Autodesk Fusion 360 part; units mm, degrees
(part 5 of 7)
  spline S32 degree 5 poles (18.221, -3.6679) (18.2206, -3.6713) (18.2199, -3.6782) (18.2192, -3.6885) (18.2187, -3.7024) (18.219, -3.7197) (18.2198, -3.7371) (18.2209, -3.7545) (18.2223, -3.7719) (18.2238, -3.7893) (18.2254, -3.8068) (18.2271, -3.8243) (18.2291, -3.8417) (18.2314, -3.8592) (18.234, -3.8768) (18.2368, -3.8943) (18.2398, -3.9118) (18.243, -3.9293) (18.2464, -3.9469) (18.2499, -3.9644) (18.2535, -3.982) (18.2574, -3.9995) (18.2614, -4.0171) (18.2655, -4.0347) (18.2699, -4.0522) (18.2744, -4.0698) (18.279, -4.0874) (18.2839, -4.1049) (18.2888, -4.1225) (18.2939, -4.1401) (18.2992, -4.1576) (18.3045, -4.1752) (18.3101, -4.1928) (18.3157, -4.2103) (18.3215, -4.2279) (18.3275, -4.2454) (18.3336, -4.2629) (18.3398, -4.2805) (18.3461, -4.298) (18.3526, -4.3155) (18.3592, -4.3331) (18.3659, -4.3506) (18.3728, -4.3681) (18.3798, -4.3856) (18.3869, -4.403) (18.3941, -4.4205) (18.4015, -4.438) (18.409, -4.4554) (18.4166, -4.4729) (18.4243, -4.4903) (18.4321, -4.5077) (18.4401, -4.5252) (18.4481, -4.5426) (18.4563, -4.5599) (18.4646, -4.5773) (18.4731, -4.5947) (18.4816, -4.612) (18.4903, -4.6293) (18.499, -4.6467) (18.5079, -4.664) (18.5169, -4.6813) (18.526, -4.6985) (18.5352, -4.7158) (18.5445, -4.733) (18.554, -4.7502) (18.5635, -4.7674) (18.5732, -4.7846) (18.5829, -4.8018) (18.5928, -4.8189) (18.6028, -4.8361) (18.6129, -4.8532) (18.621, -4.8668) (18.6272, -4.8771) (18.6313, -4.8839) (18.6334, -4.8873) knots 0 0 0 0 0 0 0.01428571 0.02857143 0.04285714 0.05714286 0.07142857 0.08571429 0.1 0.11428571 0.12857143 0.14285714 0.15714286 0.17142857 0.18571429 0.2 0.21428571 0.22857143 0.24285714 0.25714286 0.27142857 0.28571429 0.3 0.31428571 0.32857143 0.34285714 0.35714286 0.37142857 0.38571429 0.4 0.41428571 0.42857143 0.44285714 0.45714286 0.47142857 0.48571429 0.5 0.51428571 0.52857143 0.54285714 0.55714286 0.57142857 0.58571429 0.6 0.61428571 0.62857143 0.64285714 0.65714286 0.67142857 0.68571429 0.7 0.71428571 0.72857143 0.74285714 0.75714286 0.77142857 0.78571429 0.8 0.81428571 0.82857143 0.84285714 0.85714286 0.87142857 0.88571429 0.9 0.91428571 0.92857143 0.94285714 0.95714286 0.97142857 0.98571429 1 1 1 1 1 1
  arc A50 (18.6334, -4.8873) -> (19.1658, -4.8873) centre (18.8996, 2.3078) ccw
  spline S33 degree 5 poles (19.1658, -4.8873) (19.1679, -4.8839) (19.172, -4.8771) (19.1782, -4.8668) (19.1863, -4.8532) (19.1964, -4.8361) (19.2064, -4.8189) (19.2162, -4.8018) (19.226, -4.7846) (19.2356, -4.7674) (19.2452, -4.7502) (19.2546, -4.733) (19.2639, -4.7158) (19.2732, -4.6985) (19.2823, -4.6813) (19.2913, -4.664) (19.3001, -4.6467) (19.3089, -4.6293) (19.3176, -4.612) (19.3261, -4.5947) (19.3345, -4.5773) (19.3428, -4.5599) (19.351, -4.5426) (19.3591, -4.5252) (19.367, -4.5077) (19.3749, -4.4903) (19.3826, -4.4729) (19.3902, -4.4554) (19.3977, -4.438) (19.405, -4.4205) (19.4123, -4.403) (19.4194, -4.3856) (19.4264, -4.3681) (19.4332, -4.3506) (19.44, -4.3331) (19.4466, -4.3155) (19.453, -4.298) (19.4594, -4.2805) (19.4656, -4.2629) (19.4717, -4.2454) (19.4776, -4.2279) (19.4834, -4.2103) (19.4891, -4.1928) (19.4946, -4.1752) (19.5, -4.1576) (19.5052, -4.1401) (19.5103, -4.1225) (19.5153, -4.1049) (19.5201, -4.0874) (19.5248, -4.0698) (19.5293, -4.0522) (19.5336, -4.0347) (19.5378, -4.0171) (19.5418, -3.9995) (19.5456, -3.982) (19.5493, -3.9644) (19.5528, -3.9469) (19.5562, -3.9293) (19.5594, -3.9118) (19.5624, -3.8943) (19.5652, -3.8768) (19.5677, -3.8592) (19.57, -3.8417) (19.572, -3.8243) (19.5738, -3.8068) (19.5754, -3.7893) (19.5769, -3.7719) (19.5782, -3.7545) (19.5794, -3.7371) (19.5802, -3.7197) (19.5804, -3.7024) (19.58, -3.6885) (19.5793, -3.6782) (19.5786, -3.6713) (19.5782, -3.6679) knots -1 -1 -1 -1 -1 -1 -0.98571429 -0.97142857 -0.95714286 -0.94285714 -0.92857143 -0.91428571 -0.9 -0.88571429 -0.87142857 -0.85714286 -0.84285714 -0.82857143 -0.81428571 -0.8 -0.78571429 -0.77142857 -0.75714286 -0.74285714 -0.72857143 -0.71428571 -0.7 -0.68571429 -0.67142857 -0.65714286 -0.64285714 -0.62857143 -0.61428571 -0.6 -0.58571429 -0.57142857 -0.55714286 -0.54285714 -0.52857143 -0.51428571 -0.5 -0.48571429 -0.47142857 -0.45714286 -0.44285714 -0.42857143 -0.41428571 -0.4 -0.38571429 -0.37142857 -0.35714286 -0.34285714 -0.32857143 -0.31428571 -0.3 -0.28571429 -0.27142857 -0.25714286 -0.24285714 -0.22857143 -0.21428571 -0.2 -0.18571429 -0.17142857 -0.15714286 -0.14285714 -0.12857143 -0.11428571 -0.1 -0.08571429 -0.07142857 -0.05714286 -0.04285714 -0.02857143 -0.01428571 0 0 0 0 0 0
  line L50 (19.5782, -3.6679) -> (19.5395, -3.3269)
  arc A51 (19.7086, -3.1065) -> (19.5395, -3.3269) centre (19.7382, -3.3043) ccw
  line L51 (19.7086, -3.1065) -> (19.7086, -1.3065)
  line L52 (19.7086, -1.3065) -> (-29.6351, -1.3065)
  line L53 (-24.6351, -26.3065) -> (-24.6351, -3.1065)
  line L54 (-29.6351, -26.3065) -> (-24.6351, -26.3065)
  line L55 (-29.6351, -1.3065) -> (-29.6351, -26.3065)
  arc A52 (-24.466, -3.3269) -> (-24.6351, -3.1065) centre (-24.6647, -3.3043) ccw
  line L56 (-24.466, -3.3269) -> (-24.5047, -3.6679)
  spline S34 degree 5 poles (-24.5047, -3.6679) (-24.5051, -3.6713) (-24.5058, -3.6782) (-24.5065, -3.6885) (-24.5069, -3.7024) (-24.5067, -3.7197) (-24.5059, -3.7371) (-24.5047, -3.7545) (-24.5034, -3.7719) (-24.5019, -3.7893) (-24.5003, -3.8068) (-24.4985, -3.8243) (-24.4965, -3.8417) (-24.4942, -3.8592) (-24.4917, -3.8768) (-24.4889, -3.8943) (-24.4859, -3.9118) (-24.4827, -3.9293) (-24.4793, -3.9469) (-24.4758, -3.9644) (-24.4721, -3.982) (-24.4683, -3.9995) (-24.4643, -4.0171) (-24.4601, -4.0347) (-24.4558, -4.0522) (-24.4513, -4.0698) (-24.4466, -4.0874) (-24.4418, -4.1049) (-24.4368, -4.1225) (-24.4317, -4.1401) (-24.4265, -4.1576) (-24.4211, -4.1752) (-24.4156, -4.1928) (-24.4099, -4.2103) (-24.4041, -4.2279) (-24.3982, -4.2454) (-24.3921, -4.2629) (-24.3859, -4.2805) (-24.3795, -4.298) (-24.3731, -4.3155) (-24.3665, -4.3331) (-24.3597, -4.3506) (-24.3529, -4.3681) (-24.3459, -4.3856) (-24.3388, -4.403) (-24.3315, -4.4205) (-24.3242, -4.438) (-24.3167, -4.4554) (-24.3091, -4.4729) (-24.3014, -4.4903) (-24.2935, -4.5077) (-24.2856, -4.5252) (-24.2775, -4.5426) (-24.2693, -4.5599) (-24.261, -4.5773) (-24.2526, -4.5947) (-24.2441, -4.612) (-24.2354, -4.6293) (-24.2266, -4.6467) (-24.2178, -4.664) (-24.2088, -4.6813) (-24.1997, -4.6985) (-24.1904, -4.7158) (-24.1811, -4.733) (-24.1717, -4.7502) (-24.1621, -4.7674) (-24.1525, -4.7846) (-24.1427, -4.8018) (-24.1329, -4.8189) (-24.1229, -4.8361) (-24.1128, -4.8532) (-24.1047, -4.8668) (-24.0985, -4.8771) (-24.0944, -4.8839) (-24.0923, -4.8873) knots 0 0 0 0 0 0 0.01428571 0.02857143 0.04285714 0.05714286 0.07142857 0.08571429 0.1 0.11428571 0.12857143 0.14285714 0.15714286 0.17142857 0.18571429 0.2 0.21428571 0.22857143 0.24285714 0.25714286 0.27142857 0.28571429 0.3 0.31428571 0.32857143 0.34285714 0.35714286 0.37142857 0.38571429 0.4 0.41428571 0.42857143 0.44285714 0.45714286 0.47142857 0.48571429 0.5 0.51428571 0.52857143 0.54285714 0.55714286 0.57142857 0.58571429 0.6 0.61428571 0.62857143 0.64285714 0.65714286 0.67142857 0.68571429 0.7 0.71428571 0.72857143 0.74285714 0.75714286 0.77142857 0.78571429 0.8 0.81428571 0.82857143 0.84285714 0.85714286 0.87142857 0.88571429 0.9 0.91428571 0.92857143 0.94285714 0.95714286 0.97142857 0.98571429 1 1 1 1 1 1
  arc A53 (-24.0923, -4.8873) -> (-23.5599, -4.8873) centre (-23.8261, 2.3078) ccw
  spline S35 degree 5 poles (-23.5599, -4.8873) (-23.5578, -4.8839) (-23.5537, -4.8771) (-23.5475, -4.8668) (-23.5394, -4.8532) (-23.5293, -4.8361) (-23.5193, -4.8189) (-23.5094, -4.8018) (-23.4997, -4.7846) (-23.49, -4.7674) (-23.4805, -4.7502) (-23.471, -4.733) (-23.4617, -4.7158) (-23.4525, -4.6985) (-23.4434, -4.6813) (-23.4344, -4.664) (-23.4255, -4.6467) (-23.4168, -4.6293) (-23.4081, -4.612) (-23.3996, -4.5947) (-23.3911, -4.5773) (-23.3828, -4.5599) (-23.3746, -4.5426) (-23.3666, -4.5252) (-23.3586, -4.5077) (-23.3508, -4.4903) (-23.3431, -4.4729) (-23.3355, -4.4554) (-23.328, -4.438) (-23.3206, -4.4205) (-23.3134, -4.403) (-23.3063, -4.3856) (-23.2993, -4.3681) (-23.2924, -4.3506) (-23.2857, -4.3331) (-23.2791, -4.3155) (-23.2726, -4.298) (-23.2663, -4.2805) (-23.2601, -4.2629) (-23.254, -4.2454) (-23.248, -4.2279) (-23.2422, -4.2103) (-23.2366, -4.1928) (-23.231, -4.1752) (-23.2257, -4.1576) (-23.2204, -4.1401) (-23.2153, -4.1225) (-23.2104, -4.1049) (-23.2055, -4.0874) (-23.2009, -4.0698) (-23.1964, -4.0522) (-23.192, -4.0347) (-23.1879, -4.0171) (-23.1839, -3.9995) (-23.18, -3.982) (-23.1764, -3.9644) (-23.1729, -3.9469) (-23.1695, -3.9293) (-23.1663, -3.9118) (-23.1633, -3.8943) (-23.1605, -3.8768) (-23.1579, -3.8592) (-23.1556, -3.8417) (-23.1536, -3.8243) (-23.1519, -3.8068) (-23.1503, -3.7893) (-23.1488, -3.7719) (-23.1474, -3.7545) (-23.1463, -3.7371) (-23.1455, -3.7197) (-23.1452, -3.7024) (-23.1457, -3.6885) (-23.1464, -3.6782) (-23.1471, -3.6713) (-23.1475, -3.6679) knots -1 -1 -1 -1 -1 -1 -0.98571429 -0.97142857 -0.95714286 -0.94285714 -0.92857143 -0.91428571 -0.9 -0.88571429 -0.87142857 -0.85714286 -0.84285714 -0.82857143 -0.81428571 -0.8 -0.78571429 -0.77142857 -0.75714286 -0.74285714 -0.72857143 -0.71428571 -0.7 -0.68571429 -0.67142857 -0.65714286 -0.64285714 -0.62857143 -0.61428571 -0.6 -0.58571429 -0.57142857 -0.55714286 -0.54285714 -0.52857143 -0.51428571 -0.5 -0.48571429 -0.47142857 -0.45714286 -0.44285714 -0.42857143 -0.41428571 -0.4 -0.38571429 -0.37142857 -0.35714286 -0.34285714 -0.32857143 -0.31428571 -0.3 -0.28571429 -0.27142857 -0.25714286 -0.24285714 -0.22857143 -0.21428571 -0.2 -0.18571429 -0.17142857 -0.15714286 -0.14285714 -0.12857143 -0.11428571 -0.1 -0.08571429 -0.07142857 -0.05714286 -0.04285714 -0.02857143 -0.01428571 0 0 0 0 0 0
  line L57 (-23.1475, -3.6679) -> (-23.1862, -3.3269)
  line L58 (-24.6351, -3.1065) -> (-29.6351, -3.1065)
  constraint coincident L53.end A52.end
  constraint coincident L55 L58.end
  constraint perpendicular L55 L58
extrude "Extrude11" cut 1 faces at (27.9685, 26.3065, 2.0595) along direction (0, -1, 0) blind 10 on bodies 20 bodies 20
extrude "Extrude12" cut 1 faces at (27.9685, 16.3065, 2.0595) along direction (0, -1, 0) blind 2 on bodies 20 bodies 20
sketch "Sketch13" plane through (0, 0, 3.3929) normal (0, 0, 1) x (-1, 0, 0)
  line L0 (-29.6351, -14.3065) -> (-24.6351, -14.3065)
  line L1 (-24.6351, -14.3065) -> (-24.6351, -3.1065)
  arc A0 (-24.466, -3.3269) -> (-24.6351, -3.1065) centre (-24.6647, -3.3043) ccw
  line L2 (-24.466, -3.3269) -> (-24.5047, -3.6679)
  spline S0 degree 5 poles (-24.5047, -3.6679) (-24.5051, -3.6713) (-24.5058, -3.6782) (-24.5065, -3.6885) (-24.5069, -3.7024) (-24.5067, -3.7197) (-24.5059, -3.7371) (-24.5047, -3.7545) (-24.5034, -3.7719) (-24.5019, -3.7893) (-24.5003, -3.8068) (-24.4985, -3.8243) (-24.4965, -3.8417) (-24.4942, -3.8592) (-24.4917, -3.8768) (-24.4889, -3.8943) (-24.4859, -3.9118) (-24.4827, -3.9293) (-24.4793, -3.9469) (-24.4758, -3.9644) (-24.4721, -3.982) (-24.4683, -3.9995) (-24.4643, -4.0171) (-24.4601, -4.0347) (-24.4558, -4.0522) (-24.4513, -4.0698) (-24.4466, -4.0874) (-24.4418, -4.1049) (-24.4368, -4.1225) (-24.4317, -4.1401) (-24.4265, -4.1576) (-24.4211, -4.1752) (-24.4156, -4.1928) (-24.4099, -4.2103) (-24.4041, -4.2279) (-24.3982, -4.2454) (-24.3921, -4.2629) (-24.3859, -4.2805) (-24.3795, -4.298) (-24.3731, -4.3155) (-24.3665, -4.3331) (-24.3597, -4.3506) (-24.3529, -4.3681) (-24.3459, -4.3856) (-24.3388, -4.403) (-24.3315, -4.4205) (-24.3242, -4.438) (-24.3167, -4.4554) (-24.3091, -4.4729) (-24.3014, -4.4903) (-24.2935, -4.5077) (-24.2856, -4.5252) (-24.2775, -4.5426) (-24.2693, -4.5599) (-24.261, -4.5773) (-24.2526, -4.5947) (-24.2441, -4.612) (-24.2354, -4.6293) (-24.2266, -4.6467) (-24.2178, -4.664) (-24.2088, -4.6813) (-24.1997, -4.6985) (-24.1904, -4.7158) (-24.1811, -4.733) (-24.1717, -4.7502) (-24.1621, -4.7674) (-24.1525, -4.7846) (-24.1427, -4.8018) (-24.1329, -4.8189) (-24.1229, -4.8361) (-24.1128, -4.8532) (-24.1047, -4.8668) (-24.0985, -4.8771) (-24.0944, -4.8839) (-24.0923, -4.8873) knots 0 0 0 0 0 0 0.01428571 0.02857143 0.04285714 0.05714286 0.07142857 0.08571429 0.1 0.11428571 0.12857143 0.14285714 0.15714286 0.17142857 0.18571429 0.2 0.21428571 0.22857143 0.24285714 0.25714286 0.27142857 0.28571429 0.3 0.31428571 0.32857143 0.34285714 0.35714286 0.37142857 0.38571429 0.4 0.41428571 0.42857143 0.44285714 0.45714286 0.47142857 0.48571429 0.5 0.51428571 0.52857143 0.54285714 0.55714286 0.57142857 0.58571429 0.6 0.61428571 0.62857143 0.64285714 0.65714286 0.67142857 0.68571429 0.7 0.71428571 0.72857143 0.74285714 0.75714286 0.77142857 0.78571429 0.8 0.81428571 0.82857143 0.84285714 0.85714286 0.87142857 0.88571429 0.9 0.91428571 0.92857143 0.94285714 0.95714286 0.97142857 0.98571429 1 1 1 1 1 1
  arc A1 (-24.0923, -4.8873) -> (-23.5599, -4.8873) centre (-23.8261, 2.3078) ccw
  spline S1 degree 5 poles (-23.5599, -4.8873) (-23.5578, -4.8839) (-23.5537, -4.8771) (-23.5475, -4.8668) (-23.5394, -4.8532) (-23.5293, -4.8361) (-23.5193, -4.8189) (-23.5094, -4.8018) (-23.4997, -4.7846) (-23.49, -4.7674) (-23.4805, -4.7502) (-23.471, -4.733) (-23.4617, -4.7158) (-23.4525, -4.6985) (-23.4434, -4.6813) (-23.4344, -4.664) (-23.4255, -4.6467) (-23.4168, -4.6293) (-23.4081, -4.612) (-23.3996, -4.5947) (-23.3911, -4.5773) (-23.3828, -4.5599) (-23.3746, -4.5426) (-23.3666, -4.5252) (-23.3586, -4.5077) (-23.3508, -4.4903) (-23.3431, -4.4729) (-23.3355, -4.4554) (-23.328, -4.438) (-23.3206, -4.4205) (-23.3134, -4.403) (-23.3063, -4.3856) (-23.2993, -4.3681) (-23.2924, -4.3506) (-23.2857, -4.3331) (-23.2791, -4.3155) (-23.2726, -4.298) (-23.2663, -4.2805) (-23.2601, -4.2629) (-23.254, -4.2454) (-23.248, -4.2279) (-23.2422, -4.2103) (-23.2366, -4.1928) (-23.231, -4.1752) (-23.2257, -4.1576) (-23.2204, -4.1401) (-23.2153, -4.1225) (-23.2104, -4.1049) (-23.2055, -4.0874) (-23.2009, -4.0698) (-23.1964, -4.0522) (-23.192, -4.0347) (-23.1879, -4.0171) (-23.1839, -3.9995) (-23.18, -3.982) (-23.1764, -3.9644) (-23.1729, -3.9469) (-23.1695, -3.9293) (-23.1663, -3.9118) (-23.1633, -3.8943) (-23.1605, -3.8768) (-23.1579, -3.8592) (-23.1556, -3.8417) (-23.1536, -3.8243) (-23.1519, -3.8068) (-23.1503, -3.7893) (-23.1488, -3.7719) (-23.1474, -3.7545) (-23.1463, -3.7371) (-23.1455, -3.7197) (-23.1452, -3.7024) (-23.1457, -3.6885) (-23.1464, -3.6782) (-23.1471, -3.6713) (-23.1475, -3.6679) knots -1 -1 -1 -1 -1 -1 -0.98571429 -0.97142857 -0.95714286 -0.94285714 -0.92857143 -0.91428571 -0.9 -0.88571429 -0.87142857 -0.85714286 -0.84285714 -0.82857143 -0.81428571 -0.8 -0.78571429 -0.77142857 -0.75714286 -0.74285714 -0.72857143 -0.71428571 -0.7 -0.68571429 -0.67142857 -0.65714286 -0.64285714 -0.62857143 -0.61428571 -0.6 -0.58571429 -0.57142857 -0.55714286 -0.54285714 -0.52857143 -0.51428571 -0.5 -0.48571429 -0.47142857 -0.45714286 -0.44285714 -0.42857143 -0.41428571 -0.4 -0.38571429 -0.37142857 -0.35714286 -0.34285714 -0.32857143 -0.31428571 -0.3 -0.28571429 -0.27142857 -0.25714286 -0.24285714 -0.22857143 -0.21428571 -0.2 -0.18571429 -0.17142857 -0.15714286 -0.14285714 -0.12857143 -0.11428571 -0.1 -0.08571429 -0.07142857 -0.05714286 -0.04285714 -0.02857143 -0.01428571 0 0 0 0 0 0
  line L3 (-23.1475, -3.6679) -> (-23.1862, -3.3269)
  arc A2 (-23.017, -3.1065) -> (-23.1862, -3.3269) centre (-22.9875, -3.3043) ccw
  line L4 (-23.017, -3.1065) -> (-22.1219, -3.1065)
  arc A3 (-21.9527, -3.3269) -> (-22.1219, -3.1065) centre (-22.1514, -3.3043) ccw
  line L5 (-21.9527, -3.3269) -> (-21.9914, -3.6679)
  spline S2 degree 5 poles (-21.9914, -3.6679) (-21.9918, -3.6713) (-21.9925, -3.6782) (-21.9932, -3.6885) (-21.9936, -3.7024) (-21.9934, -3.7197) (-21.9926, -3.7371) (-21.9914, -3.7545) (-21.9901, -3.7719) (-21.9886, -3.7893) (-21.987, -3.8068) (-21.9852, -3.8243) (-21.9832, -3.8417) (-21.981, -3.8592) (-21.9784, -3.8768) (-21.9756, -3.8943) (-21.9726, -3.9118) (-21.9694, -3.9293) (-21.966, -3.9469) (-21.9625, -3.9644) (-21.9588, -3.982) (-21.955, -3.9995) (-21.951, -4.0171) (-21.9469, -4.0347) (-21.9425, -4.0522) (-21.938, -4.0698) (-21.9333, -4.0874) (-21.9285, -4.1049) (-21.9236, -4.1225) (-21.9185, -4.1401) (-21.9132, -4.1576) (-21.9078, -4.1752) (-21.9023, -4.1928) (-21.8966, -4.2103) (-21.8908, -4.2279) (-21.8849, -4.2454) (-21.8788, -4.2629) (-21.8726, -4.2805) (-21.8663, -4.298) (-21.8598, -4.3155) (-21.8532, -4.3331) (-21.8465, -4.3506) (-21.8396, -4.3681) (-21.8326, -4.3856) (-21.8255, -4.403) (-21.8183, -4.4205) (-21.8109, -4.438) (-21.8034, -4.4554) (-21.7958, -4.4729) (-21.7881, -4.4903) (-21.7803, -4.5077) (-21.7723, -4.5252) (-21.7642, -4.5426) (-21.7561, -4.5599) (-21.7477, -4.5773) (-21.7393, -4.5947) (-21.7308, -4.612) (-21.7221, -4.6293) (-21.7134, -4.6467) (-21.7045, -4.664) (-21.6955, -4.6813) (-21.6864, -4.6985) (-21.6772, -4.7158) (-21.6678, -4.733) (-21.6584, -4.7502) (-21.6489, -4.7674) (-21.6392, -4.7846) (-21.6295, -4.8018) (-21.6196, -4.8189) (-21.6096, -4.8361) (-21.5995, -4.8532) (-21.5914, -4.8668) (-21.5852, -4.8771) (-21.5811, -4.8839) (-21.579, -4.8873) knots 0 0 0 0 0 0 0.01428571 0.02857143 0.04285714 0.05714286 0.07142857 0.08571429 0.1 0.11428571 0.12857143 0.14285714 0.15714286 0.17142857 0.18571429 0.2 0.21428571 0.22857143 0.24285714 0.25714286 0.27142857 0.28571429 0.3 0.31428571 0.32857143 0.34285714 0.35714286 0.37142857 0.38571429 0.4 0.41428571 0.42857143 0.44285714 0.45714286 0.47142857 0.48571429 0.5 0.51428571 0.52857143 0.54285714 0.55714286 0.57142857 0.58571429 0.6 0.61428571 0.62857143 0.64285714 0.65714286 0.67142857 0.68571429 0.7 0.71428571 0.72857143 0.74285714 0.75714286 0.77142857 0.78571429 0.8 0.81428571 0.82857143 0.84285714 0.85714286 0.87142857 0.88571429 0.9 0.91428571 0.92857143 0.94285714 0.95714286 0.97142857 0.98571429 1 1 1 1 1 1
  arc A4 (-21.579, -4.8873) -> (-21.0466, -4.8873) centre (-21.3128, 2.3078) ccw
  spline S3 degree 5 poles (-21.0466, -4.8873) (-21.0445, -4.8839) (-21.0404, -4.8771) (-21.0342, -4.8668) (-21.0261, -4.8532) (-21.016, -4.8361) (-21.006, -4.8189) (-20.9962, -4.8018) (-20.9864, -4.7846) (-20.9767, -4.7674) (-20.9672, -4.7502) (-20.9578, -4.733) (-20.9484, -4.7158) (-20.9392, -4.6985) (-20.9301, -4.6813) (-20.9211, -4.664) (-20.9123, -4.6467) (-20.9035, -4.6293) (-20.8948, -4.612) (-20.8863, -4.5947) (-20.8779, -4.5773) (-20.8696, -4.5599) (-20.8614, -4.5426) (-20.8533, -4.5252) (-20.8453, -4.5077) (-20.8375, -4.4903) (-20.8298, -4.4729) (-20.8222, -4.4554) (-20.8147, -4.438) (-20.8073, -4.4205) (-20.8001, -4.403) (-20.793, -4.3856) (-20.786, -4.3681) (-20.7792, -4.3506) (-20.7724, -4.3331) (-20.7658, -4.3155) (-20.7594, -4.298) (-20.753, -4.2805) (-20.7468, -4.2629) (-20.7407, -4.2454) (-20.7348, -4.2279) (-20.729, -4.2103) (-20.7233, -4.1928) (-20.7178, -4.1752) (-20.7124, -4.1576) (-20.7071, -4.1401) (-20.702, -4.1225) (-20.6971, -4.1049) (-20.6923, -4.0874) (-20.6876, -4.0698) (-20.6831, -4.0522) (-20.6788, -4.0347) (-20.6746, -4.0171) (-20.6706, -3.9995) (-20.6668, -3.982) (-20.6631, -3.9644) (-20.6596, -3.9469) (-20.6562, -3.9293) (-20.653, -3.9118) (-20.65, -3.8943) (-20.6472, -3.8768) (-20.6446, -3.8592) (-20.6424, -3.8417) (-20.6404, -3.8243) (-20.6386, -3.8068) (-20.637, -3.7893) (-20.6355, -3.7719) (-20.6342, -3.7545) (-20.633, -3.7371) (-20.6322, -3.7197) (-20.632, -3.7024) (-20.6324, -3.6885) (-20.6331, -3.6782) (-20.6338, -3.6713) (-20.6342, -3.6679) knots -1 -1 -1 -1 -1 -1 -0.98571429 -0.97142857 -0.95714286 -0.94285714 -0.92857143 -0.91428571 -0.9 -0.88571429 -0.87142857 -0.85714286 -0.84285714 -0.82857143 -0.81428571 -0.8 -0.78571429 -0.77142857 -0.75714286 -0.74285714 -0.72857143 -0.71428571 -0.7 -0.68571429 -0.67142857 -0.65714286 -0.64285714 -0.62857143 -0.61428571 -0.6 -0.58571429 -0.57142857 -0.55714286 -0.54285714 -0.52857143 -0.51428571 -0.5 -0.48571429 -0.47142857 -0.45714286 -0.44285714 -0.42857143 -0.41428571 -0.4 -0.38571429 -0.37142857 -0.35714286 -0.34285714 -0.32857143 -0.31428571 -0.3 -0.28571429 -0.27142857 -0.25714286 -0.24285714 -0.22857143 -0.21428571 -0.2 -0.18571429 -0.17142857 -0.15714286 -0.14285714 -0.12857143 -0.11428571 -0.1 -0.08571429 -0.07142857 -0.05714286 -0.04285714 -0.02857143 -0.01428571 0 0 0 0 0 0
  line L6 (-20.6342, -3.6679) -> (-20.6729, -3.3269)
  arc A5 (-20.5037, -3.1065) -> (-20.6729, -3.3269) centre (-20.4742, -3.3043) ccw
  line L7 (-20.5037, -3.1065) -> (-19.6086, -3.1065)
  arc A6 (-19.4394, -3.3269) -> (-19.6086, -3.1065) centre (-19.6381, -3.3043) ccw
  line L8 (-19.4394, -3.3269) -> (-19.4781, -3.6679)
  spline S4 degree 5 poles (-19.4781, -3.6679) (-19.4785, -3.6713) (-19.4792, -3.6782) (-19.48, -3.6885) (-19.4804, -3.7024) (-19.4801, -3.7197) (-19.4793, -3.7371) (-19.4782, -3.7545) (-19.4768, -3.7719) (-19.4753, -3.7893) (-19.4737, -3.8068) (-19.472, -3.8243) (-19.47, -3.8417) (-19.4677, -3.8592) (-19.4652, -3.8768) (-19.4624, -3.8943) (-19.4593, -3.9118) (-19.4561, -3.9293) (-19.4528, -3.9469) (-19.4492, -3.9644) (-19.4456, -3.982) (-19.4417, -3.9995) (-19.4377, -4.0171) (-19.4336, -4.0347) (-19.4292, -4.0522) (-19.4247, -4.0698) (-19.4201, -4.0874) (-19.4153, -4.1049) (-19.4103, -4.1225) (-19.4052, -4.1401) (-19.4, -4.1576) (-19.3946, -4.1752) (-19.389, -4.1928) (-19.3834, -4.2103) (-19.3776, -4.2279) (-19.3716, -4.2454) (-19.3655, -4.2629) (-19.3593, -4.2805) (-19.353, -4.298) (-19.3465, -4.3155) (-19.3399, -4.3331) (-19.3332, -4.3506) (-19.3263, -4.3681) (-19.3193, -4.3856) (-19.3122, -4.403) (-19.305, -4.4205) (-19.2976, -4.438) (-19.2902, -4.4554) (-19.2826, -4.4729) (-19.2748, -4.4903) (-19.267, -4.5077) (-19.259, -4.5252) (-19.251, -4.5426) (-19.2428, -4.5599) (-19.2345, -4.5773) (-19.226, -4.5947) (-19.2175, -4.612) (-19.2089, -4.6293) (-19.2001, -4.6467) (-19.1912, -4.664) (-19.1822, -4.6813) (-19.1731, -4.6985) (-19.1639, -4.7158) (-19.1546, -4.733) (-19.1451, -4.7502) (-19.1356, -4.7674) (-19.1259, -4.7846) (-19.1162, -4.8018) (-19.1063, -4.8189) (-19.0963, -4.8361) (-19.0863, -4.8532) (-19.0781, -4.8668) (-19.072, -4.8771) (-19.0678, -4.8839) (-19.0658, -4.8873) knots 0 0 0 0 0 0 0.01428571 0.02857143 0.04285714 0.05714286 0.07142857 0.08571429 0.1 0.11428571 0.12857143 0.14285714 0.15714286 0.17142857 0.18571429 0.2 0.21428571 0.22857143 0.24285714 0.25714286 0.27142857 0.28571429 0.3 0.31428571 0.32857143 0.34285714 0.35714286 0.37142857 0.38571429 0.4 0.41428571 0.42857143 0.44285714 0.45714286 0.47142857 0.48571429 0.5 0.51428571 0.52857143 0.54285714 0.55714286 0.57142857 0.58571429 0.6 0.61428571 0.62857143 0.64285714 0.65714286 0.67142857 0.68571429 0.7 0.71428571 0.72857143 0.74285714 0.75714286 0.77142857 0.78571429 0.8 0.81428571 0.82857143 0.84285714 0.85714286 0.87142857 0.88571429 0.9 0.91428571 0.92857143 0.94285714 0.95714286 0.97142857 0.98571429 1 1 1 1 1 1
  arc A7 (-19.0658, -4.8873) -> (-18.5333, -4.8873) centre (-18.7995, 2.3078) ccw
  spline S5 degree 5 poles (-18.5333, -4.8873) (-18.5312, -4.8839) (-18.5271, -4.8771) (-18.521, -4.8668) (-18.5128, -4.8532) (-18.5027, -4.8361) (-18.4927, -4.8189) (-18.4829, -4.8018) (-18.4731, -4.7846) (-18.4635, -4.7674) (-18.4539, -4.7502) (-18.4445, -4.733) (-18.4352, -4.7158) (-18.426, -4.6985) (-18.4168, -4.6813) (-18.4079, -4.664) (-18.399, -4.6467) (-18.3902, -4.6293) (-18.3816, -4.612) (-18.373, -4.5947) (-18.3646, -4.5773) (-18.3563, -4.5599) (-18.3481, -4.5426) (-18.34, -4.5252) (-18.3321, -4.5077) (-18.3242, -4.4903) (-18.3165, -4.4729) (-18.3089, -4.4554) (-18.3014, -4.438) (-18.2941, -4.4205) (-18.2868, -4.403) (-18.2797, -4.3856) (-18.2727, -4.3681) (-18.2659, -4.3506) (-18.2592, -4.3331) (-18.2526, -4.3155) (-18.2461, -4.298) (-18.2397, -4.2805) (-18.2335, -4.2629) (-18.2274, -4.2454) (-18.2215, -4.2279) (-18.2157, -4.2103) (-18.21, -4.1928) (-18.2045, -4.1752) (-18.1991, -4.1576) (-18.1939, -4.1401) (-18.1888, -4.1225) (-18.1838, -4.1049) (-18.179, -4.0874) (-18.1743, -4.0698) (-18.1698, -4.0522) (-18.1655, -4.0347) (-18.1613, -4.0171) (-18.1573, -3.9995) (-18.1535, -3.982) (-18.1498, -3.9644) (-18.1463, -3.9469) (-18.1429, -3.9293) (-18.1397, -3.9118) (-18.1367, -3.8943) (-18.1339, -3.8768) (-18.1314, -3.8592) (-18.1291, -3.8417) (-18.1271, -3.8243) (-18.1253, -3.8068) (-18.1237, -3.7893) (-18.1222, -3.7719) (-18.1209, -3.7545) (-18.1197, -3.7371) (-18.1189, -3.7197) (-18.1187, -3.7024) (-18.1191, -3.6885) (-18.1198, -3.6782) (-18.1205, -3.6713) (-18.1209, -3.6679) knots -1 -1 -1 -1 -1 -1 -0.98571429 -0.97142857 -0.95714286 -0.94285714 -0.92857143 -0.91428571 -0.9 -0.88571429 -0.87142857 -0.85714286 -0.84285714 -0.82857143 -0.81428571 -0.8 -0.78571429 -0.77142857 -0.75714286 -0.74285714 -0.72857143 -0.71428571 -0.7 -0.68571429 -0.67142857 -0.65714286 -0.64285714 -0.62857143 -0.61428571 -0.6 -0.58571429 -0.57142857 -0.55714286 -0.54285714 -0.52857143 -0.51428571 -0.5 -0.48571429 -0.47142857 -0.45714286 -0.44285714 -0.42857143 -0.41428571 -0.4 -0.38571429 -0.37142857 -0.35714286 -0.34285714 -0.32857143 -0.31428571 -0.3 -0.28571429 -0.27142857 -0.25714286 -0.24285714 -0.22857143 -0.21428571 -0.2 -0.18571429 -0.17142857 -0.15714286 -0.14285714 -0.12857143 -0.11428571 -0.1 -0.08571429 -0.07142857 -0.05714286 -0.04285714 -0.02857143 -0.01428571 0 0 0 0 0 0
  line L9 (-18.1209, -3.6679) -> (-18.1596, -3.3269)
  arc A8 (-17.9905, -3.1065) -> (-18.1596, -3.3269) centre (-17.9609, -3.3043) ccw
  line L10 (-17.9905, -3.1065) -> (-17.0953, -3.1065)
  arc A9 (-16.9262, -3.3269) -> (-17.0953, -3.1065) centre (-17.1249, -3.3043) ccw
  line L11 (-16.9262, -3.3269) -> (-16.9649, -3.6679)
  spline S6 degree 5 poles (-16.9649, -3.6679) (-16.9653, -3.6713) (-16.9659, -3.6782) (-16.9667, -3.6885) (-16.9671, -3.7024) (-16.9668, -3.7197) (-16.966, -3.7371) (-16.9649, -3.7545) (-16.9635, -3.7719) (-16.9621, -3.7893) (-16.9605, -3.8068) (-16.9587, -3.8243) (-16.9567, -3.8417) (-16.9544, -3.8592) (-16.9519, -3.8768) (-16.9491, -3.8943) (-16.9461, -3.9118) (-16.9429, -3.9293) (-16.9395, -3.9469) (-16.936, -3.9644) (-16.9323, -3.982) (-16.9285, -3.9995) (-16.9245, -4.0171) (-16.9203, -4.0347) (-16.916, -4.0522) (-16.9115, -4.0698) (-16.9068, -4.0874) (-16.902, -4.1049) (-16.897, -4.1225) (-16.8919, -4.1401) (-16.8867, -4.1576) (-16.8813, -4.1752) (-16.8758, -4.1928) (-16.8701, -4.2103) (-16.8643, -4.2279) (-16.8583, -4.2454) (-16.8523, -4.2629) (-16.8461, -4.2805) (-16.8397, -4.298) (-16.8332, -4.3155) (-16.8266, -4.3331) (-16.8199, -4.3506) (-16.813, -4.3681) (-16.8061, -4.3856) (-16.799, -4.403) (-16.7917, -4.4205) (-16.7844, -4.438) (-16.7769, -4.4554) (-16.7693, -4.4729) (-16.7616, -4.4903) (-16.7537, -4.5077) (-16.7458, -4.5252) (-16.7377, -4.5426) (-16.7295, -4.5599) (-16.7212, -4.5773) (-16.7128, -4.5947) (-16.7042, -4.612) (-16.6956, -4.6293) (-16.6868, -4.6467) (-16.6779, -4.664) (-16.6689, -4.6813) (-16.6598, -4.6985) (-16.6506, -4.7158) (-16.6413, -4.733) (-16.6319, -4.7502) (-16.6223, -4.7674) (-16.6127, -4.7846) (-16.6029, -4.8018) (-16.593, -4.8189) (-16.5831, -4.8361) (-16.573, -4.8532) (-16.5648, -4.8668) (-16.5587, -4.8771) (-16.5545, -4.8839) (-16.5525, -4.8873) knots 0 0 0 0 0 0 0.01428571 0.02857143 0.04285714 0.05714286 0.07142857 0.08571429 0.1 0.11428571 0.12857143 0.14285714 0.15714286 0.17142857 0.18571429 0.2 0.21428571 0.22857143 0.24285714 0.25714286 0.27142857 0.28571429 0.3 0.31428571 0.32857143 0.34285714 0.35714286 0.37142857 0.38571429 0.4 0.41428571 0.42857143 0.44285714 0.45714286 0.47142857 0.48571429 0.5 0.51428571 0.52857143 0.54285714 0.55714286 0.57142857 0.58571429 0.6 0.61428571 0.62857143 0.64285714 0.65714286 0.67142857 0.68571429 0.7 0.71428571 0.72857143 0.74285714 0.75714286 0.77142857 0.78571429 0.8 0.81428571 0.82857143 0.84285714 0.85714286 0.87142857 0.88571429 0.9 0.91428571 0.92857143 0.94285714 0.95714286 0.97142857 0.98571429 1 1 1 1 1 1
  arc A10 (-16.5525, -4.8873) -> (-16.02, -4.8873) centre (-16.2863, 2.3078) ccw
  spline S7 degree 5 poles (-16.02, -4.8873) (-16.018, -4.8839) (-16.0138, -4.8771) (-16.0077, -4.8668) (-15.9995, -4.8532) (-15.9894, -4.8361) (-15.9795, -4.8189) (-15.9696, -4.8018) (-15.9598, -4.7846) (-15.9502, -4.7674) (-15.9407, -4.7502) (-15.9312, -4.733) (-15.9219, -4.7158) (-15.9127, -4.6985) (-15.9036, -4.6813) (-15.8946, -4.664) (-15.8857, -4.6467) (-15.8769, -4.6293) (-15.8683, -4.612) (-15.8597, -4.5947) (-15.8513, -4.5773) (-15.843, -4.5599) (-15.8348, -4.5426) (-15.8267, -4.5252) (-15.8188, -4.5077) (-15.811, -4.4903) (-15.8032, -4.4729) (-15.7956, -4.4554) (-15.7882, -4.438) (-15.7808, -4.4205) (-15.7736, -4.403) (-15.7665, -4.3856) (-15.7595, -4.3681) (-15.7526, -4.3506) (-15.7459, -4.3331) (-15.7393, -4.3155) (-15.7328, -4.298) (-15.7265, -4.2805) (-15.7202, -4.2629) (-15.7142, -4.2454) (-15.7082, -4.2279) (-15.7024, -4.2103) (-15.6967, -4.1928) (-15.6912, -4.1752) (-15.6858, -4.1576) (-15.6806, -4.1401) (-15.6755, -4.1225) (-15.6705, -4.1049) (-15.6657, -4.0874) (-15.6611, -4.0698) (-15.6565, -4.0522) (-15.6522, -4.0347) (-15.648, -4.0171) (-15.644, -3.9995) (-15.6402, -3.982) (-15.6365, -3.9644) (-15.633, -3.9469) (-15.6297, -3.9293) (-15.6265, -3.9118) (-15.6234, -3.8943) (-15.6206, -3.8768) (-15.6181, -3.8592) (-15.6158, -3.8417) (-15.6138, -3.8243) (-15.612, -3.8068) (-15.6104, -3.7893) (-15.609, -3.7719) (-15.6076, -3.7545) (-15.6065, -3.7371) (-15.6057, -3.7197) (-15.6054, -3.7024) (-15.6058, -3.6885) (-15.6066, -3.6782) (-15.6073, -3.6713) (-15.6076, -3.6679) knots -1 -1 -1 -1 -1 -1 -0.98571429 -0.97142857 -0.95714286 -0.94285714 -0.92857143 -0.91428571 -0.9 -0.88571429 -0.87142857 -0.85714286 -0.84285714 -0.82857143 -0.81428571 -0.8 -0.78571429 -0.77142857 -0.75714286 -0.74285714 -0.72857143 -0.71428571 -0.7 -0.68571429 -0.67142857 -0.65714286 -0.64285714 -0.62857143 -0.61428571 -0.6 -0.58571429 -0.57142857 -0.55714286 -0.54285714 -0.52857143 -0.51428571 -0.5 -0.48571429 -0.47142857 -0.45714286 -0.44285714 -0.42857143 -0.41428571 -0.4 -0.38571429 -0.37142857 -0.35714286 -0.34285714 -0.32857143 -0.31428571 -0.3 -0.28571429 -0.27142857 -0.25714286 -0.24285714 -0.22857143 -0.21428571 -0.2 -0.18571429 -0.17142857 -0.15714286 -0.14285714 -0.12857143 -0.11428571 -0.1 -0.08571429 -0.07142857 -0.05714286 -0.04285714 -0.02857143 -0.01428571 0 0 0 0 0 0
  line L12 (-15.6076, -3.6679) -> (-15.6464, -3.3269)
  arc A11 (-15.4772, -3.1065) -> (-15.6464, -3.3269) centre (-15.4476, -3.3043) ccw
  line L13 (-15.4772, -3.1065) -> (-14.582, -3.1065)
  arc A12 (-14.4129, -3.3269) -> (-14.582, -3.1065) centre (-14.6116, -3.3043) ccw
  line L14 (-14.4129, -3.3269) -> (-14.4516, -3.6679)
  spline S8 degree 5 poles (-14.4516, -3.6679) (-14.452, -3.6713) (-14.4527, -3.6782) (-14.4534, -3.6885) (-14.4538, -3.7024) (-14.4536, -3.7197) (-14.4528, -3.7371) (-14.4516, -3.7545) (-14.4503, -3.7719) (-14.4488, -3.7893) (-14.4472, -3.8068) (-14.4454, -3.8243) (-14.4434, -3.8417) (-14.4411, -3.8592) (-14.4386, -3.8768) (-14.4358, -3.8943) (-14.4328, -3.9118) (-14.4296, -3.9293) (-14.4262, -3.9469) (-14.4227, -3.9644) (-14.419, -3.982) (-14.4152, -3.9995) (-14.4112, -4.0171) (-14.407, -4.0347) (-14.4027, -4.0522) (-14.3982, -4.0698) (-14.3935, -4.0874) (-14.3887, -4.1049) (-14.3837, -4.1225) (-14.3786, -4.1401) (-14.3734, -4.1576) (-14.368, -4.1752) (-14.3625, -4.1928) (-14.3568, -4.2103) (-14.351, -4.2279) (-14.3451, -4.2454) (-14.339, -4.2629) (-14.3328, -4.2805) (-14.3264, -4.298) (-14.32, -4.3155) (-14.3134, -4.3331) (-14.3066, -4.3506) (-14.2998, -4.3681) (-14.2928, -4.3856) (-14.2857, -4.403) (-14.2784, -4.4205) (-14.2711, -4.438) (-14.2636, -4.4554) (-14.256, -4.4729) (-14.2483, -4.4903) (-14.2405, -4.5077) (-14.2325, -4.5252) (-14.2244, -4.5426) (-14.2162, -4.5599) (-14.2079, -4.5773) (-14.1995, -4.5947) (-14.191, -4.612) (-14.1823, -4.6293) (-14.1735, -4.6467) (-14.1647, -4.664) (-14.1557, -4.6813) (-14.1466, -4.6985) (-14.1374, -4.7158) (-14.128, -4.733) (-14.1186, -4.7502) (-14.109, -4.7674) (-14.0994, -4.7846) (-14.0896, -4.8018) (-14.0798, -4.8189) (-14.0698, -4.8361) (-14.0597, -4.8532) (-14.0516, -4.8668) (-14.0454, -4.8771) (-14.0413, -4.8839) (-14.0392, -4.8873) knots 0 0 0 0 0 0 0.01428571 0.02857143 0.04285714 0.05714286 0.07142857 0.08571429 0.1 0.11428571 0.12857143 0.14285714 0.15714286 0.17142857 0.18571429 0.2 0.21428571 0.22857143 0.24285714 0.25714286 0.27142857 0.28571429 0.3 0.31428571 0.32857143 0.34285714 0.35714286 0.37142857 0.38571429 0.4 0.41428571 0.42857143 0.44285714 0.45714286 0.47142857 0.48571429 0.5 0.51428571 0.52857143 0.54285714 0.55714286 0.57142857 0.58571429 0.6 0.61428571 0.62857143 0.64285714 0.65714286 0.67142857 0.68571429 0.7 0.71428571 0.72857143 0.74285714 0.75714286 0.77142857 0.78571429 0.8 0.81428571 0.82857143 0.84285714 0.85714286 0.87142857 0.88571429 0.9 0.91428571 0.92857143 0.94285714 0.95714286 0.97142857 0.98571429 1 1 1 1 1 1
  arc A13 (-14.0392, -4.8873) -> (-13.5068, -4.8873) centre (-13.773, 2.3078) ccw
  spline S9 degree 5 poles (-13.5068, -4.8873) (-13.5047, -4.8839) (-13.5006, -4.8771) (-13.4944, -4.8668) (-13.4863, -4.8532) (-13.4762, -4.8361) (-13.4662, -4.8189) (-13.4563, -4.8018) (-13.4466, -4.7846) (-13.4369, -4.7674) (-13.4274, -4.7502) (-13.4179, -4.733) (-13.4086, -4.7158) (-13.3994, -4.6985) (-13.3903, -4.6813) (-13.3813, -4.664) (-13.3724, -4.6467) (-13.3637, -4.6293) (-13.355, -4.612) (-13.3465, -4.5947) (-13.338, -4.5773) (-13.3297, -4.5599) (-13.3215, -4.5426) (-13.3135, -4.5252) (-13.3055, -4.5077) (-13.2977, -4.4903) (-13.29, -4.4729) (-13.2824, -4.4554) (-13.2749, -4.438) (-13.2675, -4.4205) (-13.2603, -4.403) (-13.2532, -4.3856) (-13.2462, -4.3681) (-13.2393, -4.3506) (-13.2326, -4.3331) (-13.226, -4.3155) (-13.2195, -4.298) (-13.2132, -4.2805) (-13.207, -4.2629) (-13.2009, -4.2454) (-13.1949, -4.2279) (-13.1891, -4.2103) (-13.1835, -4.1928) (-13.1779, -4.1752) (-13.1726, -4.1576) (-13.1673, -4.1401) (-13.1622, -4.1225) (-13.1573, -4.1049) (-13.1524, -4.0874) (-13.1478, -4.0698) (-13.1433, -4.0522) (-13.1389, -4.0347) (-13.1348, -4.0171) (-13.1308, -3.9995) (-13.1269, -3.982) (-13.1233, -3.9644) (-13.1198, -3.9469) (-13.1164, -3.9293) (-13.1132, -3.9118) (-13.1102, -3.8943) (-13.1074, -3.8768) (-13.1048, -3.8592) (-13.1025, -3.8417) (-13.1005, -3.8243) (-13.0988, -3.8068) (-13.0972, -3.7893) (-13.0957, -3.7719) (-13.0944, -3.7545) (-13.0932, -3.7371) (-13.0924, -3.7197) (-13.0921, -3.7024) (-13.0926, -3.6885) (-13.0933, -3.6782) (-13.094, -3.6713) (-13.0944, -3.6679) knots -1 -1 -1 -1 -1 -1 -0.98571429 -0.97142857 -0.95714286 -0.94285714 -0.92857143 -0.91428571 -0.9 -0.88571429 -0.87142857 -0.85714286 -0.84285714 -0.82857143 -0.81428571 -0.8 -0.78571429 -0.77142857 -0.75714286 -0.74285714 -0.72857143 -0.71428571 -0.7 -0.68571429 -0.67142857 -0.65714286 -0.64285714 -0.62857143 -0.61428571 -0.6 -0.58571429 -0.57142857 -0.55714286 -0.54285714 -0.52857143 -0.51428571 -0.5 -0.48571429 -0.47142857 -0.45714286 -0.44285714 -0.42857143 -0.41428571 -0.4 -0.38571429 -0.37142857 -0.35714286 -0.34285714 -0.32857143 -0.31428571 -0.3 -0.28571429 -0.27142857 -0.25714286 -0.24285714 -0.22857143 -0.21428571 -0.2 -0.18571429 -0.17142857 -0.15714286 -0.14285714 -0.12857143 -0.11428571 -0.1 -0.08571429 -0.07142857 -0.05714286 -0.04285714 -0.02857143 -0.01428571 0 0 0 0 0 0
  line L15 (-13.0944, -3.6679) -> (-13.1331, -3.3269)
  arc A14 (-12.9639, -3.1065) -> (-13.1331, -3.3269) centre (-12.9344, -3.3043) ccw
  line L16 (-12.9639, -3.1065) -> (-12.0688, -3.1065)
  arc A15 (-11.8996, -3.3269) -> (-12.0688, -3.1065) centre (-12.0983, -3.3043) ccw
  line L17 (-11.8996, -3.3269) -> (-11.9383, -3.6679)
  spline S10 degree 5 poles (-11.9383, -3.6679) (-11.9387, -3.6713) (-11.9394, -3.6782) (-11.9401, -3.6885) (-11.9405, -3.7024) (-11.9403, -3.7197) (-11.9395, -3.7371) (-11.9383, -3.7545) (-11.937, -3.7719) (-11.9355, -3.7893) (-11.9339, -3.8068) (-11.9321, -3.8243) (-11.9301, -3.8417) (-11.9279, -3.8592) (-11.9253, -3.8768) (-11.9225, -3.8943) (-11.9195, -3.9118) (-11.9163, -3.9293) (-11.9129, -3.9469) (-11.9094, -3.9644) (-11.9058, -3.982) (-11.9019, -3.9995) (-11.8979, -4.0171) (-11.8938, -4.0347) (-11.8894, -4.0522) (-11.8849, -4.0698) (-11.8802, -4.0874) (-11.8754, -4.1049) (-11.8705, -4.1225) (-11.8654, -4.1401) (-11.8601, -4.1576) (-11.8547, -4.1752) (-11.8492, -4.1928) (-11.8436, -4.2103) (-11.8377, -4.2279) (-11.8318, -4.2454) (-11.8257, -4.2629) (-11.8195, -4.2805) (-11.8132, -4.298) (-11.8067, -4.3155) (-11.8001, -4.3331) (-11.7934, -4.3506) (-11.7865, -4.3681) (-11.7795, -4.3856) (-11.7724, -4.403) (-11.7652, -4.4205) (-11.7578, -4.438) (-11.7503, -4.4554) (-11.7427, -4.4729) (-11.735, -4.4903) (-11.7272, -4.5077) (-11.7192, -4.5252) (-11.7111, -4.5426) (-11.703, -4.5599) (-11.6946, -4.5773) (-11.6862, -4.5947) (-11.6777, -4.612) (-11.669, -4.6293) (-11.6603, -4.6467) (-11.6514, -4.664) (-11.6424, -4.6813) (-11.6333, -4.6985) (-11.6241, -4.7158) (-11.6148, -4.733) (-11.6053, -4.7502) (-11.5958, -4.7674) (-11.5861, -4.7846) (-11.5764, -4.8018) (-11.5665, -4.8189) (-11.5565, -4.8361) (-11.5464, -4.8532) (-11.5383, -4.8668) (-11.5321, -4.8771) (-11.528, -4.8839) (-11.5259, -4.8873) knots 0 0 0 0 0 0 0.01428571 0.02857143 0.04285714 0.05714286 0.07142857 0.08571429 0.1 0.11428571 0.12857143 0.14285714 0.15714286 0.17142857 0.18571429 0.2 0.21428571 0.22857143 0.24285714 0.25714286 0.27142857 0.28571429 0.3 0.31428571 0.32857143 0.34285714 0.35714286 0.37142857 0.38571429 0.4 0.41428571 0.42857143 0.44285714 0.45714286 0.47142857 0.48571429 0.5 0.51428571 0.52857143 0.54285714 0.55714286 0.57142857 0.58571429 0.6 0.61428571 0.62857143 0.64285714 0.65714286 0.67142857 0.68571429 0.7 0.71428571 0.72857143 0.74285714 0.75714286 0.77142857 0.78571429 0.8 0.81428571 0.82857143 0.84285714 0.85714286 0.87142857 0.88571429 0.9 0.91428571 0.92857143 0.94285714 0.95714286 0.97142857 0.98571429 1 1 1 1 1 1
  arc A16 (-11.5259, -4.8873) -> (-10.9935, -4.8873) centre (-11.2597, 2.3078) ccw
  spline S11 degree 5 poles (-10.9935, -4.8873) (-10.9914, -4.8839) (-10.9873, -4.8771) (-10.9811, -4.8668) (-10.973, -4.8532) (-10.9629, -4.8361) (-10.9529, -4.8189) (-10.9431, -4.8018) (-10.9333, -4.7846) (-10.9236, -4.7674) (-10.9141, -4.7502) (-10.9047, -4.733) (-10.8953, -4.7158) (-10.8861, -4.6985) (-10.877, -4.6813) (-10.868, -4.664) (-10.8592, -4.6467) (-10.8504, -4.6293) (-10.8417, -4.612) (-10.8332, -4.5947) (-10.8248, -4.5773) (-10.8165, -4.5599) (-10.8083, -4.5426) (-10.8002, -4.5252) (-10.7922, -4.5077) (-10.7844, -4.4903) (-10.7767, -4.4729) (-10.7691, -4.4554) (-10.7616, -4.438) (-10.7542, -4.4205) (-10.747, -4.403) (-10.7399, -4.3856) (-10.7329, -4.3681) (-10.7261, -4.3506) (-10.7193, -4.3331) (-10.7127, -4.3155) (-10.7063, -4.298) (-10.6999, -4.2805) (-10.6937, -4.2629) (-10.6876, -4.2454) (-10.6817, -4.2279) (-10.6759, -4.2103) (-10.6702, -4.1928) (-10.6647, -4.1752) (-10.6593, -4.1576) (-10.654, -4.1401) (-10.6489, -4.1225) (-10.644, -4.1049) (-10.6392, -4.0874) (-10.6345, -4.0698) (-10.63, -4.0522) (-10.6257, -4.0347) (-10.6215, -4.0171) (-10.6175, -3.9995) (-10.6137, -3.982) (-10.61, -3.9644) (-10.6065, -3.9469) (-10.6031, -3.9293) (-10.5999, -3.9118) (-10.5969, -3.8943) (-10.5941, -3.8768) (-10.5915, -3.8592) (-10.5893, -3.8417) (-10.5873, -3.8243) (-10.5855, -3.8068) (-10.5839, -3.7893) (-10.5824, -3.7719) (-10.5811, -3.7545) (-10.5799, -3.7371) (-10.5791, -3.7197) (-10.5789, -3.7024) (-10.5793, -3.6885) (-10.58, -3.6782) (-10.5807, -3.6713) (-10.5811, -3.6679) knots -1 -1 -1 -1 -1 -1 -0.98571429 -0.97142857 -0.95714286 -0.94285714 -0.92857143 -0.91428571 -0.9 -0.88571429 -0.87142857 -0.85714286 -0.84285714 -0.82857143 -0.81428571 -0.8 -0.78571429 -0.77142857 -0.75714286 -0.74285714 -0.72857143 -0.71428571 -0.7 -0.68571429 -0.67142857 -0.65714286 -0.64285714 -0.62857143 -0.61428571 -0.6 -0.58571429 -0.57142857 -0.55714286 -0.54285714 -0.52857143 -0.51428571 -0.5 -0.48571429 -0.47142857 -0.45714286 -0.44285714 -0.42857143 -0.41428571 -0.4 -0.38571429 -0.37142857 -0.35714286 -0.34285714 -0.32857143 -0.31428571 -0.3 -0.28571429 -0.27142857 -0.25714286 -0.24285714 -0.22857143 -0.21428571 -0.2 -0.18571429 -0.17142857 -0.15714286 -0.14285714 -0.12857143 -0.11428571 -0.1 -0.08571429 -0.07142857 -0.05714286 -0.04285714 -0.02857143 -0.01428571 0 0 0 0 0 0
  line L18 (-10.5811, -3.6679) -> (-10.6198, -3.3269)
  arc A17 (-10.4507, -3.1065) -> (-10.6198, -3.3269) centre (-10.4211, -3.3043) ccw
  line L19 (-10.4507, -3.1065) -> (-9.5555, -3.1065)
  arc A18 (-9.3863, -3.3269) -> (-9.5555, -3.1065) centre (-9.5851, -3.3043) ccw
  line L20 (-9.3863, -3.3269) -> (-9.425, -3.6679)
  spline S12 degree 5 poles (-9.425, -3.6679) (-9.4254, -3.6713) (-9.4261, -3.6782) (-9.4269, -3.6885) (-9.4273, -3.7024) (-9.427, -3.7197) (-9.4262, -3.7371) (-9.4251, -3.7545) (-9.4237, -3.7719) (-9.4223, -3.7893) (-9.4207, -3.8068) (-9.4189, -3.8243) (-9.4169, -3.8417) (-9.4146, -3.8592) (-9.4121, -3.8768) (-9.4093, -3.8943) (-9.4062, -3.9118) (-9.403, -3.9293) (-9.3997, -3.9469) (-9.3961, -3.9644) (-9.3925, -3.982) (-9.3886, -3.9995) (-9.3847, -4.0171) (-9.3805, -4.0347) (-9.3761, -4.0522) (-9.3716, -4.0698) (-9.367, -4.0874) (-9.3622, -4.1049) (-9.3572, -4.1225) (-9.3521, -4.1401) (-9.3469, -4.1576) (-9.3415, -4.1752) (-9.3359, -4.1928) (-9.3303, -4.2103) (-9.3245, -4.2279) (-9.3185, -4.2454) (-9.3124, -4.2629) (-9.3062, -4.2805) (-9.2999, -4.298) (-9.2934, -4.3155) (-9.2868, -4.3331) (-9.2801, -4.3506) (-9.2732, -4.3681) (-9.2662, -4.3856) (-9.2591, -4.403) (-9.2519, -4.4205) (-9.2445, -4.438) (-9.2371, -4.4554) (-9.2295, -4.4729) (-9.2217, -4.4903) (-9.2139, -4.5077) (-9.2059, -4.5252) (-9.1979, -4.5426) (-9.1897, -4.5599) (-9.1814, -4.5773) (-9.1729, -4.5947) (-9.1644, -4.612) (-9.1558, -4.6293) (-9.147, -4.6467) (-9.1381, -4.664) (-9.1291, -4.6813) (-9.12, -4.6985) (-9.1108, -4.7158) (-9.1015, -4.733) (-9.092, -4.7502) (-9.0825, -4.7674) (-9.0728, -4.7846) (-9.0631, -4.8018) (-9.0532, -4.8189) (-9.0432, -4.8361) (-9.0332, -4.8532) (-9.025, -4.8668) (-9.0189, -4.8771) (-9.0147, -4.8839) (-9.0127, -4.8873) knots 0 0 0 0 0 0 0.01428571 0.02857143 0.04285714 0.05714286 0.07142857 0.08571429 0.1 0.11428571 0.12857143 0.14285714 0.15714286 0.17142857 0.18571429 0.2 0.21428571 0.22857143 0.24285714 0.25714286 0.27142857 0.28571429 0.3 0.31428571 0.32857143 0.34285714 0.35714286 0.37142857 0.38571429 0.4 0.41428571 0.42857143 0.44285714 0.45714286 0.47142857 0.48571429 0.5 0.51428571 0.52857143 0.54285714 0.55714286 0.57142857 0.58571429 0.6 0.61428571 0.62857143 0.64285714 0.65714286 0.67142857 0.68571429 0.7 0.71428571 0.72857143 0.74285714 0.75714286 0.77142857 0.78571429 0.8 0.81428571 0.82857143 0.84285714 0.85714286 0.87142857 0.88571429 0.9 0.91428571 0.92857143 0.94285714 0.95714286 0.97142857 0.98571429 1 1 1 1 1 1
  arc A19 (-9.0127, -4.8873) -> (-8.4802, -4.8873) centre (-8.7464, 2.3078) ccw
  spline S13 degree 5 poles (-8.4802, -4.8873) (-8.4781, -4.8839) (-8.474, -4.8771) (-8.4679, -4.8668) (-8.4597, -4.8532) (-8.4496, -4.8361) (-8.4397, -4.8189) (-8.4298, -4.8018) (-8.42, -4.7846) (-8.4104, -4.7674) (-8.4008, -4.7502) (-8.3914, -4.733) (-8.3821, -4.7158) (-8.3729, -4.6985) (-8.3638, -4.6813) (-8.3548, -4.664) (-8.3459, -4.6467) (-8.3371, -4.6293) (-8.3285, -4.612) (-8.3199, -4.5947) (-8.3115, -4.5773) (-8.3032, -4.5599) (-8.295, -4.5426) (-8.2869, -4.5252) (-8.279, -4.5077) (-8.2711, -4.4903) (-8.2634, -4.4729) (-8.2558, -4.4554) (-8.2483, -4.438) (-8.241, -4.4205) (-8.2337, -4.403) (-8.2266, -4.3856) (-8.2196, -4.3681) (-8.2128, -4.3506) (-8.2061, -4.3331) (-8.1995, -4.3155) (-8.193, -4.298) (-8.1866, -4.2805) (-8.1804, -4.2629) (-8.1743, -4.2454) (-8.1684, -4.2279) (-8.1626, -4.2103) (-8.1569, -4.1928) (-8.1514, -4.1752) (-8.146, -4.1576) (-8.1408, -4.1401) (-8.1357, -4.1225) (-8.1307, -4.1049) (-8.1259, -4.0874) (-8.1212, -4.0698) (-8.1167, -4.0522) (-8.1124, -4.0347) (-8.1082, -4.0171) (-8.1042, -3.9995) (-8.1004, -3.982) (-8.0967, -3.9644) (-8.0932, -3.9469) (-8.0898, -3.9293) (-8.0866, -3.9118) (-8.0836, -3.8943) (-8.0808, -3.8768) (-8.0783, -3.8592) (-8.076, -3.8417) (-8.074, -3.8243) (-8.0722, -3.8068) (-8.0706, -3.7893) (-8.0691, -3.7719) (-8.0678, -3.7545) (-8.0667, -3.7371) (-8.0658, -3.7197) (-8.0656, -3.7024) (-8.066, -3.6885) (-8.0667, -3.6782) (-8.0674, -3.6713) (-8.0678, -3.6679) knots -1 -1 -1 -1 -1 -1 -0.98571429 -0.97142857 -0.95714286 -0.94285714 -0.92857143 -0.91428571 -0.9 -0.88571429 -0.87142857 -0.85714286 -0.84285714 -0.82857143 -0.81428571 -0.8 -0.78571429 -0.77142857 -0.75714286 -0.74285714 -0.72857143 -0.71428571 -0.7 -0.68571429 -0.67142857 -0.65714286 -0.64285714 -0.62857143 -0.61428571 -0.6 -0.58571429 -0.57142857 -0.55714286 -0.54285714 -0.52857143 -0.51428571 -0.5 -0.48571429 -0.47142857 -0.45714286 -0.44285714 -0.42857143 -0.41428571 -0.4 -0.38571429 -0.37142857 -0.35714286 -0.34285714 -0.32857143 -0.31428571 -0.3 -0.28571429 -0.27142857 -0.25714286 -0.24285714 -0.22857143 -0.21428571 -0.2 -0.18571429 -0.17142857 -0.15714286 -0.14285714 -0.12857143 -0.11428571 -0.1 -0.08571429 -0.07142857 -0.05714286 -0.04285714 -0.02857143 -0.01428571 0 0 0 0 0 0
  line L21 (-8.0678, -3.6679) -> (-8.1065, -3.3269)
  arc A20 (-7.9374, -3.1065) -> (-8.1065, -3.3269) centre (-7.9078, -3.3043) ccw
  line L22 (-7.9374, -3.1065) -> (-7.0422, -3.1065)
  arc A21 (-6.8731, -3.3269) -> (-7.0422, -3.1065) centre (-7.0718, -3.3043) ccw
  line L23 (-6.8731, -3.3269) -> (-6.9118, -3.6679)
  spline S14 degree 5 poles (-6.9118, -3.6679) (-6.9122, -3.6713) (-6.9128, -3.6782) (-6.9136, -3.6885) (-6.914, -3.7024) (-6.9138, -3.7197) (-6.9129, -3.7371) (-6.9118, -3.7545) (-6.9105, -3.7719) (-6.909, -3.7893) (-6.9074, -3.8068) (-6.9056, -3.8243) (-6.9036, -3.8417) (-6.9013, -3.8592) (-6.8988, -3.8768) (-6.896, -3.8943) (-6.893, -3.9118) (-6.8898, -3.9293) (-6.8864, -3.9469) (-6.8829, -3.9644) (-6.8792, -3.982) (-6.8754, -3.9995) (-6.8714, -4.0171) (-6.8672, -4.0347) (-6.8629, -4.0522) (-6.8584, -4.0698) (-6.8537, -4.0874) (-6.8489, -4.1049) (-6.8439, -4.1225) (-6.8388, -4.1401) (-6.8336, -4.1576) (-6.8282, -4.1752) (-6.8227, -4.1928) (-6.817, -4.2103) (-6.8112, -4.2279) (-6.8053, -4.2454) (-6.7992, -4.2629) (-6.793, -4.2805) (-6.7866, -4.298) (-6.7801, -4.3155) (-6.7735, -4.3331) (-6.7668, -4.3506) (-6.76, -4.3681) (-6.753, -4.3856) (-6.7459, -4.403) (-6.7386, -4.4205) (-6.7313, -4.438) (-6.7238, -4.4554) (-6.7162, -4.4729) (-6.7085, -4.4903) (-6.7006, -4.5077) (-6.6927, -4.5252) (-6.6846, -4.5426) (-6.6764, -4.5599) (-6.6681, -4.5773) (-6.6597, -4.5947) (-6.6511, -4.612) (-6.6425, -4.6293) (-6.6337, -4.6467) (-6.6248, -4.664) (-6.6158, -4.6813) (-6.6067, -4.6985) (-6.5975, -4.7158) (-6.5882, -4.733) (-6.5788, -4.7502) (-6.5692, -4.7674) (-6.5596, -4.7846) (-6.5498, -4.8018) (-6.5399, -4.8189) (-6.53, -4.8361) (-6.5199, -4.8532) (-6.5117, -4.8668) (-6.5056, -4.8771) (-6.5015, -4.8839) (-6.4994, -4.8873) knots 0 0 0 0 0 0 0.01428571 0.02857143 0.04285714 0.05714286 0.07142857 0.08571429 0.1 0.11428571 0.12857143 0.14285714 0.15714286 0.17142857 0.18571429 0.2 0.21428571 0.22857143 0.24285714 0.25714286 0.27142857 0.28571429 0.3 0.31428571 0.32857143 0.34285714 0.35714286 0.37142857 0.38571429 0.4 0.41428571 0.42857143 0.44285714 0.45714286 0.47142857 0.48571429 0.5 0.51428571 0.52857143 0.54285714 0.55714286 0.57142857 0.58571429 0.6 0.61428571 0.62857143 0.64285714 0.65714286 0.67142857 0.68571429 0.7 0.71428571 0.72857143 0.74285714 0.75714286 0.77142857 0.78571429 0.8 0.81428571 0.82857143 0.84285714 0.85714286 0.87142857 0.88571429 0.9 0.91428571 0.92857143 0.94285714 0.95714286 0.97142857 0.98571429 1 1 1 1 1 1
  arc A22 (-6.4994, -4.8873) -> (-5.9669, -4.8873) centre (-6.2332, 2.3078) ccw
  spline S15 degree 5 poles (-5.9669, -4.8873) (-5.9649, -4.8839) (-5.9607, -4.8771) (-5.9546, -4.8668) (-5.9464, -4.8532) (-5.9364, -4.8361) (-5.9264, -4.8189) (-5.9165, -4.8018) (-5.9067, -4.7846) (-5.8971, -4.7674) (-5.8876, -4.7502) (-5.8781, -4.733) (-5.8688, -4.7158) (-5.8596, -4.6985) (-5.8505, -4.6813) (-5.8415, -4.664) (-5.8326, -4.6467) (-5.8238, -4.6293) (-5.8152, -4.612) (-5.8067, -4.5947) (-5.7982, -4.5773) (-5.7899, -4.5599) (-5.7817, -4.5426) (-5.7737, -4.5252) (-5.7657, -4.5077) (-5.7579, -4.4903) (-5.7501, -4.4729) (-5.7425, -4.4554) (-5.7351, -4.438) (-5.7277, -4.4205) (-5.7205, -4.403) (-5.7134, -4.3856) (-5.7064, -4.3681) (-5.6995, -4.3506) (-5.6928, -4.3331) (-5.6862, -4.3155) (-5.6797, -4.298) (-5.6734, -4.2805) (-5.6672, -4.2629) (-5.6611, -4.2454) (-5.6551, -4.2279) (-5.6493, -4.2103) (-5.6437, -4.1928) (-5.6381, -4.1752) (-5.6327, -4.1576) (-5.6275, -4.1401) (-5.6224, -4.1225) (-5.6174, -4.1049) (-5.6126, -4.0874) (-5.608, -4.0698) (-5.6035, -4.0522) (-5.5991, -4.0347) (-5.5949, -4.0171) (-5.5909, -3.9995) (-5.5871, -3.982) (-5.5835, -3.9644) (-5.5799, -3.9469) (-5.5766, -3.9293) (-5.5734, -3.9118) (-5.5703, -3.8943) (-5.5675, -3.8768) (-5.565, -3.8592) (-5.5627, -3.8417) (-5.5607, -3.8243) (-5.5589, -3.8068) (-5.5573, -3.7893) (-5.5559, -3.7719) (-5.5545, -3.7545) (-5.5534, -3.7371) (-5.5526, -3.7197) (-5.5523, -3.7024) (-5.5527, -3.6885) (-5.5535, -3.6782) (-5.5542, -3.6713) (-5.5545, -3.6679) knots -1 -1 -1 -1 -1 -1 -0.98571429 -0.97142857 -0.95714286 -0.94285714 -0.92857143 -0.91428571 -0.9 -0.88571429 -0.87142857 -0.85714286 -0.84285714 -0.82857143 -0.81428571 -0.8 -0.78571429 -0.77142857 -0.75714286 -0.74285714 -0.72857143 -0.71428571 -0.7 -0.68571429 -0.67142857 -0.65714286 -0.64285714 -0.62857143 -0.61428571 -0.6 -0.58571429 -0.57142857 -0.55714286 -0.54285714 -0.52857143 -0.51428571 -0.5 -0.48571429 -0.47142857 -0.45714286 -0.44285714 -0.42857143 -0.41428571 -0.4 -0.38571429 -0.37142857 -0.35714286 -0.34285714 -0.32857143 -0.31428571 -0.3 -0.28571429 -0.27142857 -0.25714286 -0.24285714 -0.22857143 -0.21428571 -0.2 -0.18571429 -0.17142857 -0.15714286 -0.14285714 -0.12857143 -0.11428571 -0.1 -0.08571429 -0.07142857 -0.05714286 -0.04285714 -0.02857143 -0.01428571 0 0 0 0 0 0
  line L24 (-5.5545, -3.6679) -> (-5.5933, -3.3269)
  arc A23 (-5.4241, -3.1065) -> (-5.5933, -3.3269) centre (-5.3945, -3.3043) ccw
  line L25 (-5.4241, -3.1065) -> (-4.5289, -3.1065)
  arc A24 (-4.3598, -3.3269) -> (-4.5289, -3.1065) centre (-4.5585, -3.3043) ccw
  line L26 (-4.3598, -3.3269) -> (-4.3985, -3.6679)